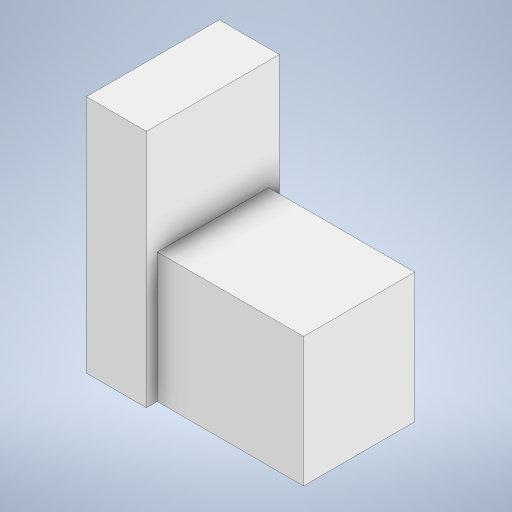
# Autodesk Inventor part: Toilet
Saved by Autodesk Inventor 2024 (Build 280153000, 153)
## iProperties
Created: 2023-05-15
Part Number: Toilet
Material: Steel
Document SubType Name: Modeling
Designer: Tom
Density: 7.85 g/cm^3
Appearance: White
Mass: 1.15838e+06 g
Surface Area: 19748.1 cm^2
Volume: 147565 cm^3
Author: Tom
Autodesk Inventor part; units mm, degrees
ref_plane "YZ Plane" through (0, 0, 0) normal (1, 0, 0) x (0, 1, 0)
ref_plane "XZ Plane" through (0, 0, 0) normal (0, 1, 0) x (-1, 0, 0)
ref_plane "XY Plane" through (0, 0, 0) normal (0, 0, 1) x (1, 0, 0)
sketch "Sketch1" plane through (0, 0, 0) normal (1, 0, 0) x (0, 1, 0)
  line L0 (0, 0) -> (795.02, 0)
  line L1 (795.02, 0) -> (795.02, -441.96)
  line L2 (795.02, -441.96) -> (0, -441.96)
  line L3 (0, -441.96) -> (0, 0)
  dimension "d1" = 441.96
  dimension "d2" = 795.02
  constraints: 8 end point, 2 parallel, 1 horizontal, 1 perpendicular
  measures "d1" distance of L0.end L1.end
  measures "d2" distance of L0.start L0.end
extrude "Extrusion1" add sketch "Sketch1" along normal blind 199.898
sketch "Sketch2" plane through (199.898, 0, 0) normal (1, 0, 0) x (0, 0, -1)
  line L0 (0, 0) -> (441.96, 0) projected
  line L1 (35.941, 0) -> (406.019, 0)
  line L2 (406.019, 0) -> (406.019, 430.022)
  line L3 (406.019, 430.022) -> (35.941, 430.022)
  line L4 (35.941, 430.022) -> (35.941, 0)
  line L5 (0, 795.02) -> (0, 0) projected
  dimension "d5" = 370.078
  dimension "d6" = 430.022
  dimension "d7" = 35.941
  constraints: 8 end point, 2 parallel, 1 horizontal, 1 perpendicular, 1 point on line
  measures "d5" distance of L2.end L3.end
  measures "d6" distance of L1.end L2.end
  measures "d7" distance between parallel lines of L5 L4
extrude "Extrusion2" add sketch "Sketch2" along normal blind 485.902
body "Solid1"
